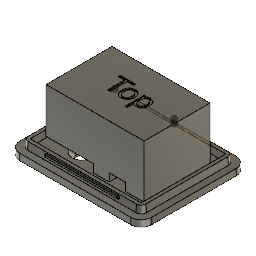
ESP8266 Relay Board Case (Autodesk Fusion 360 design; units mm, degrees)
Autodesk Fusion 360 part; units mm, degrees
note: some values were not read from the file. Chosen so that the rebuilt part matches the saved one: which bodies a step acts on; which face or edge a step refers to; the sign of a taper; the layout of a text; where a step ends.
sketch "Sketch1" plane through (0, 0, 0) normal (0, 0, 1) x (1, 0, 0)
  line L0 (-25, 20) -> (25, 20)
  line L1 (25, 20) -> (25, -20)
  line L2 (25, -20) -> (-25, -20)
  line L3 (-25, -20) -> (-25, 20)
  line L4 (-25, 20) -> (25, -20) construction
  line L5 (25, 20) -> (-25, -20) construction
  dimension "d1" = 50
  dimension "d2" = 40
  constraint perpendicular L0 L1
  constraint parallel L0 L2
  constraint parallel L1 L3
  constraint horizontal L0
  constraint coincident L4 origin
  constraint coincident L5 origin
  measures "d1" distance of L1.end L2.end
  measures "d2" distance of L0.end L1.end
  measures "d80" distance of L0.end
extrude "Extrude1" add sketch "Sketch1" along normal blind 30 makes body 1
fillet "Fillet1" radius 4 8 edges at (-25, -20, 15) (0, -20, 30) (25, -20, 15) (25, 20, 15) (25, 0, 30) (0, 20, 30) (-25, 20, 15) (-25, 0, 30) on bodies 1
copy_body "Body->Comp1" bodies 1 removing the originals makes body 2 in component "Component"
ref_plane "WorkPlane1" through (0, 0, 2.5) normal (0, 0, -1) x (-1, 0, 0)
split "Split1" by plane through (0, 0, 2.5) normal (0, 0, -1) bodies 2 makes body 3 at (7, -6.6667, 0) in component "Component"
sketch "Sketch1 (2)" plane through (0, 0, 0) normal (0, 0, 1) x (1, 0, 0) in component "ESP8266"
  line L0 (-18.6, 12.5) -> (18.6, 12.5)
  line L1 (18.6, 12.5) -> (18.6, -12.5)
  line L2 (18.6, -12.5) -> (-18.6, -12.5)
  line L3 (-18.6, -12.5) -> (-18.6, 12.5)
  line L4 (-18.6, 12.5) -> (18.6, -12.5) construction
  line L5 (18.6, 12.5) -> (-18.6, -12.5) construction
  dimension "d7" = 37.2
  dimension "d8" = 25
  constraint perpendicular L0 L1
  constraint parallel L0 L2
  constraint parallel L1 L3
  constraint horizontal L0
  constraint coincident L4 origin
  constraint coincident L5 origin
  measures "d7" distance of L1.end L2.end
  measures "d8" distance of L0.end L1.end
extrude "Extrude1'" add sketch "Sketch1 (2)" along normal blind 20 separate body makes body 4 in component "ESP8266"
sketch "Sketch2" plane through (-18.6, 0, 0) normal (-1, 0, 0) x (0, -1, 0) in component "ESP8266"
  line L0 (-12.5, 0) -> (12.5, 0)
  line L1 (12.5, 0) -> (12.5, 20)
  line L2 (12.5, 20) -> (-12.5, 20)
  line L3 (-12.5, 20) -> (-12.5, 0)
  line L4 (-0.5, 7.5) -> (3.5, 7.5)
  line L5 (3.5, 7.5) -> (3.5, 4)
  line L6 (3.5, 4) -> (-0.5, 4)
  line L7 (-0.5, 4) -> (-0.5, 7.5)
  dimension "d11" = 9
  dimension "d12" = 4
  dimension "d13" = 4
  dimension "d14" = 3.5
  constraint horizontal L4
  constraint vertical L5
  constraint horizontal L6
  constraint vertical L7
  measures "d11" distance of L1 L5.end
  measures "d12" distance of L5.end L6.end
  measures "d13" distance of L0 L6
  measures "d14" distance of L4.end L5.end
extrude "Extrude2" add sketch "Sketch2" along normal blind 3.4 contours L4 L5 L6 L7 bodies 4 in component "ESP8266"
sketch "Sketch3" plane through (0, 0, 20) normal (0, 0, 1) x (-1, 0, 0) in component "ESP8266"
  line L0 (18.6, 12.5) -> (-18.6, 12.5)
  line L1 (-18.6, 12.5) -> (-18.6, -12.5)
  line L2 (-18.6, -12.5) -> (18.6, -12.5)
  line L3 (18.6, -12.5) -> (18.6, 12.5)
  line L4 (7.4649, 4.5924) -> (-8.0234, 4.5924) construction
  line L5 (-8.0234, 4.5924) -> (-8.0234, -5.4076) construction
  line L6 (-8.0234, -5.4076) -> (7.4649, -5.4076) construction
  line L7 (7.4649, -5.4076) -> (7.4649, 4.5924) construction
  text T0 "Top" font "Arial" height 10 align ink ink in box 0 x 0 at (7.4549, 4.5724) x (-1, 0) y (0, -1) spacing 1 kerned height is em
  constraint perpendicular L4 L5
  constraint parallel L4 L6
  constraint parallel L5 L7
extrude "Extrude3" cut sketch "Sketch3" against normal blind 0.423 text T0 bodies 4 in component "ESP8266"
shell "Shell1" thickness 4 removed faces 1 at (-7, -6.6667, 2.5) on bodies 2 in component "Component"
sketch "Sketch1 (3)" plane through (-25, 0, 0) normal (-1, 0, 0) x (0, -1, 0) in component "Component"
  line L0 (-16, 2.5) -> (16, 2.5)
  line L1 (16, 2.5) -> (16, 26)
  line L2 (16, 26) -> (-16, 26)
  line L3 (-16, 26) -> (-16, 2.5)
  line L4 (-0.5, 6.5) -> (-0.5, 10)
  line L5 (-0.5, 10) -> (3.5, 10)
  line L6 (3.5, 10) -> (3.5, 6.5)
  line L7 (3.5, 6.5) -> (-0.5, 6.5)
  line L8 (-12.5, 2.5) -> (12.5, 2.5)
  line L9 (12.5, 2.5) -> (12.5, 22.5)
  line L10 (12.5, 22.5) -> (-12.5, 22.5)
  line L11 (-12.5, 22.5) -> (-12.5, 2.5)
  line L12 (-0.5, 10) -> (3.5, 6.5) construction
  circle A0 centre (1.5, 8.25) radius 3.5
  dimension "d32" = 7
  constraint coincident L4.end L5.start
  constraint coincident L6.end L7.start
  constraint midpoint L12 A0.centre
  measures "d32" diameter of A0
extrude "Extrude1''" cut sketch "Sketch1 (3)" along normal up to far side of body 4 placed x (1, 0, 0) y (0, 1, 0) z (0, 0, 1) at (0, 0, 2.5) contours L4 L5 L6 L7 | A0 bodies 2 in component "Component"
sketch "Sketch2 (2)" plane through (0, 0, 2.5) normal (0, 0, -1) x (1, 0, 0) in component "Component"
  line L0 (-21, -16) -> (-21, 16)
  line L1 (-21, 16) -> (21, 16)
  line L2 (21, 16) -> (21, -16)
  line L3 (21, -16) -> (-21, -16)
  arc A0 (-21, 20) -> (-25, 16) centre (-21, 16) ccw
  line L4 (-25, 16) -> (-25, -16)
  arc A1 (-25, -16) -> (-21, -20) centre (-21, -16) ccw
  line L5 (-21, -20) -> (21, -20)
  arc A2 (21, -20) -> (25, -16) centre (21, -16) ccw
  line L6 (25, -16) -> (25, 16)
  arc A3 (25, 16) -> (21, 20) centre (21, 16) ccw
  line L7 (21, 20) -> (-21, 20)
  line L8 (-22.5, -17.5) -> (-22.5, 17.5)
  line L9 (-22.5, 17.5) -> (22.5, 17.5)
  line L10 (22.5, 17.5) -> (22.5, -17.5)
  line L11 (22.5, -17.5) -> (-22.5, -17.5)
  dimension "d36" = -1.5
extrude "Extrude2'" cut sketch "Sketch2 (2)" against normal blind 3 contours L8 L9 L10 L11 bodies 2 in component "Component"
sketch "Sketch3 (2)" plane through (0, 17.5, 0) normal (0, -1, 0) x (1, 0, 0) in component "Component"
  line L0 (-22.5, 2.5) -> (22.5, 2.5)
  line L1 (22.5, 2.5) -> (22.5, 5.5)
  line L2 (22.5, 5.5) -> (-22.5, 5.5)
  line L3 (-22.5, 5.5) -> (-22.5, 2.5)
  line L4 (-14, 4.5) -> (14, 4.5)
  line L5 (14, 4.5) -> (14, 3.5)
  line L6 (14, 3.5) -> (-14, 3.5)
  line L7 (-14, 3.5) -> (-14, 4.5)
  line L8 (-14, 4.5) -> (14, 3.5) construction
  point P0 (0, 4)
  point P1 (0, 5.5)
  point P2 (-22.5, 4)
  dimension "d39" = 28
  dimension "d40" = 1
  constraint horizontal L4
  constraint vertical L5
  constraint horizontal L6
  constraint vertical L7
  constraint midpoint L8 P0
  constraint midpoint L2 P1
  constraint midpoint L3 P2
  constraint vertical P0 P1
  constraint horizontal P0 P2
  measures "d39" distance of L4.start L4.end
  measures "d40" distance of L4.start L6.end
extrude "Extrude3'" cut sketch "Sketch3 (2)" against normal blind 1 draft -45 contours L4 L5 L6 L7 bodies 2 in component "Component"
ref_plane "WorkPlane1" through (0, 0, 14.25) normal (0, -1, 0) x (1, 0, 0) in component "Component"
mirror "Mirror1" about plane through (0, 0, 14.25) normal (0, -1, 0) of "Extrude3'" in component "Component"
sketch "Sketch4" plane through (0, 0, 2.5) normal (0, 0, 1) x (-1, 0, 0) in component "Component"
  arc A0 (25, 16) -> (21, 20) centre (21, 16) ccw
  line L0 (21, 20) -> (-21, 20)
  arc A1 (-21, 20) -> (-25, 16) centre (-21, 16) ccw
  line L1 (-25, 16) -> (-25, -16)
  arc A2 (-25, -16) -> (-21, -20) centre (-21, -16) ccw
  line L2 (-21, -20) -> (21, -20)
  arc A3 (21, -20) -> (25, -16) centre (21, -16) ccw
  line L3 (25, -16) -> (25, 16)
  line L4 (-21, 16) -> (-21, -16)
  line L5 (-21, -16) -> (21, -16)
  line L6 (21, -16) -> (21, -0.6651)
  line L7 (21, -0.6651) -> (22.5, -0.6651)
  line L8 (22.5, -0.6651) -> (22.5, -17.5)
  line L9 (22.5, -17.5) -> (-22.5, -17.5)
  line L10 (-22.5, -17.5) -> (-22.5, 17.5)
  line L11 (-22.5, 17.5) -> (22.5, 17.5)
  line L12 (22.5, 17.5) -> (22.5, 3.6651)
  line L13 (22.5, 3.6651) -> (21, 3.6651)
  line L14 (21, 3.6651) -> (21, 16)
  line L15 (21, 16) -> (-21, 16)
extrude "Extrude4" add sketch "Sketch4" along normal blind 2.7 contours L4 L5 L6 L7 L8 L9 L10 L11 L12 L13 L14 L15 bodies 3 in component "Component"
extrude "Extrude5" add sketch "Sketch3 (2)" against normal blind 1 draft -45 contours L4 L5 L6 L7 bodies 3 in component "Component"
mirror "Mirror2" about plane through (0, 0, 14.25) normal (0, -1, 0) of "Extrude5" in component "Component"
fillet "Fillet1'" radius 2 4 edges at (-22.5, 17.5, 3.85) (-22.5, -17.5, 3.85) (22.5, 17.5, 3.85) (22.5, -17.5, 3.85) on bodies 3 in component "Component"
draft "Draft1" angle -5 neutral plane through (0, 0, 2.5) pull (0, 0, -1) 9 faces at (-18.3333, -17.5, 3.7333) (20.5952, -17.4977, 3.4) (22.5, 5.1667, 4.3) (21.5, 17.2321, 3.4) (-18.3333, 17.5, 3.7333) (-20.6901, 17.4909, 3.4) (-22.5, 5.61, 3.4) (-22.3567, -16.2433, 3.4) (-22.5, -7.61, 4.3) on bodies 3 in component "Component"
sketch "Sketch4 (2)" plane through (0, 0, 0) normal (0, 0, -1) x (1, 0, 0) in component "ESP8266"
  line L0 (18.6, 12.5) -> (-18.6, 12.5)
  line L1 (-18.6, 12.5) -> (-18.6, -12.5)
  line L2 (-18.6, -12.5) -> (18.6, -12.5)
  line L3 (18.6, -12.5) -> (18.6, 12.5)
  line L4 (-18.6, -6.5) -> (18.6, -6.5)
  line L5 (-18.6, 6) -> (-14.6, 6)
  line L6 (-14.6, 6) -> (-14.6, -3)
  line L7 (-14.6, -3) -> (-18.6, -3)
  line L8 (-18.6, -3) -> (-18.6, 6)
  line L9 (-0.6, 12.5) -> (-0.6, -6.5)
  line L10 (5.4, 12.5) -> (5.4, -6.5)
  line L11 (11.6, 12.5) -> (11.6, -6.5)
  dimension "d52" = 6
  dimension "d53" = 9
  dimension "d54" = 4
  dimension "d55" = 9.5
  dimension "d57" = 6
  dimension "d58" = 18
  dimension "d59" = 7
  constraint coincident L1 L4.start
  constraint coincident L3 L4.end
  constraint horizontal L4
  constraint horizontal L5
  constraint vertical L6
  constraint horizontal L7
  constraint vertical L8
  constraint coincident L1 L5.start
  constraint coincident L0 L9.start
  constraint coincident L4 L9.end
  constraint perpendicular L4 L9
  constraint coincident L0 L10.start
  constraint coincident L4 L10.end
  constraint perpendicular L4 L10
  constraint coincident L0 L11.start
  constraint coincident L4 L11.end
  constraint perpendicular L4 L11
  measures "d52" distance of L2 L4
  measures "d53" distance of L5.start L7.end
  measures "d54" distance of L5.start L5.end
  measures "d55" distance of L2 L7
  measures "d57" distance of L9 L10
  measures "d58" distance of L1 L9
  measures "d59" distance of L3 L11
extrude "Extrude4'" cut sketch "Sketch4 (2)" against normal blind 3 contours L0 L4 L10 L11 | L0 L1 L4 L5 L6 L7 L9 bodies 4 in component "ESP8266"
sketch "Sketch6" plane through (0, 0, 2.5) normal (0, 0, 1) x (-1, 0, 0) in component "Component"
  line L0 (22.5, 3.6651) -> (21, 3.6651)
  line L1 (21, 3.6651) -> (21, 16)
  line L2 (21, 16) -> (-21, 16)
  line L3 (-21, 16) -> (-21, -16)
  line L4 (-21, -16) -> (21, -16)
  line L5 (21, -16) -> (21, -0.6651)
  line L6 (21, -0.6651) -> (22.5, -0.6651)
  line L7 (22.5, -0.6651) -> (22.5, -15.5)
  arc A0 (20.5, -17.5) -> (22.5, -15.5) centre (20.5, -15.5) ccw
  line L8 (20.5, -17.5) -> (-20.5, -17.5)
  arc A1 (-22.5, -15.5) -> (-20.5, -17.5) centre (-20.5, -15.5) ccw
  line L9 (-22.5, -15.5) -> (-22.5, 15.5)
  arc A2 (-20.5, 17.5) -> (-22.5, 15.5) centre (-20.5, 15.5) ccw
  line L10 (-20.5, 17.5) -> (20.5, 17.5)
  arc A3 (22.5, 15.5) -> (20.5, 17.5) centre (20.5, 15.5) ccw
  line L11 (22.5, 15.5) -> (22.5, 3.6651)
  line L12 (25, -16) -> (25, 16)
  arc A4 (25, 16) -> (21, 20) centre (21, 16) ccw
  line L13 (21, 20) -> (-21, 20)
  arc A5 (-21, 20) -> (-25, 16) centre (-21, 16) ccw
  line L14 (-25, 16) -> (-25, -16)
  arc A6 (-25, -16) -> (-21, -20) centre (-21, -16) ccw
  line L15 (-21, -20) -> (21, -20)
  arc A7 (21, -20) -> (25, -16) centre (21, -16) ccw
  line L16 (18.6, 12.5) -> (18.6, 6)
  line L17 (18.6, 6) -> (14.6, 6)
  line L18 (14.6, 6) -> (14.6, -3)
  line L19 (14.6, -3) -> (18.6, -3)
  line L20 (18.6, -3) -> (18.6, -6.5)
  line L21 (18.6, -6.5) -> (0.6, -6.5)
  line L22 (0.6, -6.5) -> (0.6, 12.5)
  line L23 (0.6, 12.5) -> (18.6, 12.5)
  circle A8 centre (9.6, 8) radius 2
  circle A9 centre (-8.7, 4) radius 2
  circle A10 centre (-8.7, 4) radius 3.6 construction
  circle A11 centre (9.6, 8) radius 3.6 construction
  dimension "d62" = 4
  dimension "d64" = 7.2
  dimension "d67" = 4.5
  dimension "d68" = 9
  dimension "d74" = 27.3
  dimension "d75" = 8.5
  constraint concentric A9 A10
  constraint concentric A8 A11
  constraint equal A8 A9
  constraint equal A10 A11
  measures "d62" diameter of A8
  measures "d64" diameter of A10
  measures "d67" distance of L23 A8.centre
  measures "d68" horizontal distance of L16.start A8.centre
  measures "d74" horizontal distance of L16.start A9.centre
  measures "d75" vertical distance of L16.start A9.centre
hole "Hole1" at (8.7, -4, 2.5) at (-9.6, -8, 2.5) direction (0, 0, -1) diameter 3.7 depth 8 tip angle 118 countersink diameter 7.144 countersink angle 90 bodies 3 in component "Component"
fillet "Fillet2" radius 0.5 1 edges at (0, -18, 4) on bodies 3 in component "Component"
fillet "Fillet2" radius 0.5 4 edges at (-13.8459, -17.6541, 4.3459) (-13.7902, -17.7098, 3.7098) (13.8459, -17.6541, 4.3459) (13.7902, -17.7098, 3.7098) on bodies 3 in component "Component"
fillet "Fillet2" radius 0.5 5 edges at (13.8459, 17.6541, 4.3459) (13.7902, 17.7098, 3.7098) (0, 18, 4) (-13.7902, 17.7098, 3.7098) (-13.8459, 17.6541, 4.3459) on bodies 3 in component "Component"
sketch "Sketch7" plane through (0, 20, 0) normal (0, 1, 0) x (-1, 0, 0) in component "Component"
  line L0 (-21, 2.5) -> (21, 2.5)
  line L1 (21, 2.5) -> (21, 26)
  line L2 (21, 26) -> (-21, 26)
  line L3 (-21, 26) -> (-21, 2.5)
  line L4 (-18.6, 11.5) -> (3.4, 11.5)
  line L5 (3.4, 11.5) -> (3.4, 2.5)
  line L6 (3.4, 2.5) -> (-18.6, 2.5)
  line L7 (-18.6, 2.5) -> (-18.6, 11.5)
  line L8 (-18.6, 2.5) -> (-18.6, 22.5)
  dimension "d79" = 22
  dimension "d80" = 9
  constraint horizontal L4
  constraint vertical L5
  constraint horizontal L6
  constraint vertical L7
  constraint collinear L0 L6
  constraint coincident L4.start L8
  measures "d79" distance of L4.start L4.end
  measures "d80" distance of L4.start L6.end
extrude "Extrude6" cut sketch "Sketch7" against normal blind 2.5 contours L0 L4 L5 L6 L7 L8 bodies 2 in component "Component"
fillet "Fillet3" radius 3 2 edges at (-3.4, 18.75, 11.5) (18.6, 18.75, 11.5) on bodies 2 in component "Component"
component "ESP8266" placed x (1, 0, 0) y (0, 1, 0) z (0, 0, 1) at (0, 0, 2.5)
component "Component" placed x (1, 0, 0) y (0, 1, 0) z (0, 0, 1) at (0, 0, 0)
hidden bodies 2
named bodies: "Cap", "Base"
